Autodesk Fusion 360 part; units mm, degrees
note: some values were not read from the file. Set by a fixed rule: which face or edge a step refers to.
(part 4 of 4)
sketch "Sketch106" plane through (-154.276, 154.276, 0) normal (0.707107, -0.707107, 0) x (0.707107, 0.707107, 0)
  line L0 (-683.7427, -256.3488) -> (-383.7427, -256.3488)
  line L1 (-383.7427, -256.3488) -> (-383.7427, 273.6512)
  line L2 (-383.7427, 273.6512) -> (-683.7427, 273.6512)
  line L3 (-683.7427, 273.6512) -> (-683.7427, -256.3488)
  line L4 (-451.5546, -67.3925) -> (-616.5546, -67.3925)
  line L5 (-616.5546, -67.3925) -> (-616.5546, 97.6075)
  line L6 (-616.5546, 97.6075) -> (-451.5546, 97.6075)
  line L7 (-451.5546, 97.6075) -> (-451.5546, -67.3925)
  line L8 (-634.0546, 115.1075) -> (-434.0546, 115.1075)
  line L9 (-434.0546, 115.1075) -> (-434.0546, -84.8925)
  line L10 (-434.0546, -84.8925) -> (-634.0546, -84.8925)
  line L11 (-634.0546, -84.8925) -> (-634.0546, 115.1075)
  dimension "d553" = 200
  dimension "d554" = 200
  constraint horizontal L8
  constraint vertical L9
  constraint horizontal L10
  constraint vertical L11
  measures "d553" distance of L8.start L8.end
  measures "d554" distance of L8.start L10.end
extrude "Extrude70" cut sketch "Sketch106" against normal blind 10 contours L8 L9 L10 L11 bodies 9
sketch "Sketch107" plane through (0, -41, 0) normal (0, -1, 0) x (1, 0, 0)
  circle A0 centre (-282.6941, 15.6014) radius 82.5
  line L0 (-412.6941, -83.8986) -> (-392.6941, -103.8986)
  line L1 (-392.6941, -103.8986) -> (-172.6941, -103.8986)
  line L2 (-172.6941, -103.8986) -> (-152.6941, -83.8986)
  line L3 (-152.6941, -83.8986) -> (-152.6941, 116.1014)
  line L4 (-152.6941, 116.1014) -> (-172.6941, 136.1014)
  line L5 (-172.6941, 136.1014) -> (-392.6941, 136.1014)
  line L6 (-392.6941, 136.1014) -> (-412.6941, 116.1014)
  line L7 (-412.6941, 116.1014) -> (-412.6941, -83.8986)
  line L8 (-367.6941, 101.1014) -> (-197.6941, 101.1014)
  line L9 (-197.6941, 101.1014) -> (-197.6941, -68.8986)
  line L10 (-197.6941, -68.8986) -> (-367.6941, -68.8986)
  line L11 (-367.6941, -68.8986) -> (-367.6941, 101.1014)
  dimension "d557" = 170
  dimension "d558" = 170
  constraint horizontal L8
  constraint vertical L9
  constraint horizontal L10
  constraint vertical L11
  measures "d557" distance of L8.start L8.end
  measures "d558" distance of L8.start L10.end
extrude "Extrude71" add sketch "Sketch107" along normal blind 0.1 separate body contours A0 | L8 L9 L10 L11 makes body 34
sketch "Sketch108" plane through (0, -41, 0) normal (0, -1, 0) x (1, 0, 0)
sketch "Sketch109" plane through (0, -41, 0) normal (0, -1, 0) x (1, 0, 0)
  line L0 (-375.6941, -61.8986) -> (-367.6941, -61.8986)
  line L1 (-360.6941, -68.8986) -> (-360.6941, -76.8986)
  line L2 (-360.6941, -76.8986) -> (-375.6941, -76.8986)
  line L3 (-375.6941, -76.8986) -> (-375.6941, -61.8986)
  line L4 (-197.6941, -61.8986) -> (-189.6941, -61.8986)
  line L5 (-189.6941, -61.8986) -> (-189.6941, -76.8986)
  line L6 (-189.6941, -76.8986) -> (-204.6941, -76.8986)
  line L7 (-204.6941, -76.8986) -> (-204.6941, -68.8986)
  line L8 (-360.6941, -68.8986) -> (-367.6941, -68.8986)
  line L9 (-367.6941, -68.8986) -> (-367.6941, -61.8986)
  line L10 (-197.6941, -61.8986) -> (-197.6941, -68.8986)
  line L11 (-197.6941, -68.8986) -> (-204.6941, -68.8986)
  circle A0 centre (-193.6941, -72.8986) radius 2
  circle A1 centre (-371.6941, -72.8986) radius 2
  point P0 (-367.6941, -68.8986)
  point P1 (-197.6941, -68.8986)
  dimension "d568" = 15
  dimension "d573" = 7
  dimension "d576" = 4
  dimension "d577" = 4
  constraint horizontal L0
  constraint vertical L1
  constraint horizontal L2
  constraint vertical L3
  constraint horizontal L4
  constraint vertical L5
  constraint horizontal L6
  constraint vertical L7
  constraint horizontal L8
  constraint vertical L9
  constraint vertical L10
  constraint horizontal L11
  constraint coincident P0 L8.end
  constraint coincident P1 L10.end
  measures "d568" distance of L0.start L2.end
  measures "d573" distance of L0.end P0
  measures "d576" diameter of A0
  measures "d577" diameter of A1
extrude "Extrude72" add sketch "Sketch109" along normal blind 3 separate body makes body 35 at (-363.0274, -41, -71.5653) makes body 36 at (-202.3608, -41, -71.5653)
sketch "Sketch110" plane through (0, -38, 0) normal (0, 1, 0) x (-1, 0, 0)
sketch "Sketch111" plane through (0, -41, 0) normal (0, -1, 0) x (1, 0, 0)
  circle A0 centre (-371.6941, -72.8986) radius 2
  circle A1 centre (-193.7228, -72.9066) radius 2
  point P0 (-375.6941, -76.8986)
  point P1 (-189.6941, -76.8986)
  dimension "d580" = 4
  dimension "d581" = 4
  measures "d580" diameter of A0
  measures "d581" diameter of A1
sketch "Sketch112" plane through (0, -41, 0) normal (0, -1, 0) x (1, 0, 0)
sketch "Sketch113" plane through (0, -41, 0) normal (0, -1, 0) x (1, 0, 0)
sketch "Sketch114" plane through (0, -41, 0) normal (0, -1, 0) x (1, 0, 0)
extrude "Extrude73" cut sketch "Sketch111" against normal blind 3 bodies 30
sketch "Sketch115" plane through (0, 0, 273.1014) normal (0, 0, 1) x (-1, 0, 0)
  arc A0 (177.6941, 0) -> (172.6941, 0) centre (175.1941, 0) ccw
  line L0 (177.6941, 0) -> (197.6941, 0)
  arc A1 (202.6941, 0) -> (197.6941, 0) centre (200.1941, 0) ccw
  line L1 (202.6941, 0) -> (202.6941, -10)
  line L2 (202.6941, -10) -> (362.6941, -10)
  line L3 (362.6941, -10) -> (362.6941, 0)
  arc A2 (367.694, 0) -> (362.6941, 0) centre (365.1941, 0.0132) ccw
  line L4 (367.694, 0) -> (387.6941, 0)
  arc A3 (392.6941, 0) -> (387.6941, 0) centre (390.1941, 0) ccw
  line L5 (392.6941, 0) -> (392.6941, -10)
  line L6 (392.6941, -10) -> (422.6941, -10)
  line L7 (422.6941, -10) -> (422.6941, 25)
  arc A4 (422.6941, 30) -> (422.6941, 25) centre (422.6941, 27.5) ccw
  line L8 (422.6941, 30) -> (432.6941, 30)
  line L9 (432.6941, 30) -> (432.6941, 60)
  line L10 (432.6941, 60) -> (422.6941, 60)
  arc A5 (422.6941, 65) -> (422.6941, 60) centre (422.6941, 62.5) ccw
  line L11 (422.6941, 65) -> (422.6941, 100)
  line L12 (422.6941, 100) -> (142.6941, 100)
  line L13 (142.6941, 100) -> (142.6941, 65)
  arc A6 (142.6941, 60) -> (142.6941, 65) centre (142.6941, 62.5) ccw
  line L14 (142.6941, 60) -> (132.6941, 60)
  line L15 (132.6941, 60) -> (132.6941, 30)
  line L16 (132.6941, 30) -> (142.6941, 30)
  arc A7 (142.6941, 25) -> (142.6941, 30) centre (142.6941, 27.5) ccw
  line L17 (142.6941, 25) -> (142.6941, -10)
  line L18 (142.6941, -10) -> (172.6941, -10)
  line L19 (172.6941, -10) -> (172.6941, 0)
  circle A8 centre (400.1941, 22.3451) radius 12.5
sketch "Sketch116" plane through (0, 0, -256.8986) normal (0, 0, -1) x (1, 0, 0)
  line L0 (-332.6941, 30) -> (-332.6941, 80)
  line L1 (-332.6941, 80) -> (-232.6941, 80)
  line L2 (-232.6941, 80) -> (-232.6941, 30)
  line L3 (-232.6941, 30) -> (-332.6941, 30)
  arc A0 (-172.6941, 0) -> (-177.6941, 0) centre (-175.1941, 0) ccw
  line L4 (-172.6941, 0) -> (-172.6941, -10)
  line L5 (-172.6941, -10) -> (-142.6941, -10)
  line L6 (-142.6941, -10) -> (-142.6941, 25)
  arc A1 (-142.6941, 30) -> (-142.6941, 25) centre (-142.6941, 27.5) ccw
  line L7 (-142.6941, 30) -> (-132.6941, 30)
  line L8 (-132.6941, 30) -> (-132.6941, 60)
  line L9 (-132.6941, 60) -> (-142.6941, 60)
  arc A2 (-142.6941, 65) -> (-142.6941, 60) centre (-142.6941, 62.5) ccw
  line L10 (-142.6941, 65) -> (-142.6941, 100)
  line L11 (-142.6941, 100) -> (-422.6941, 100)
  line L12 (-422.6941, 100) -> (-422.6941, 65)
  arc A3 (-422.6941, 60) -> (-422.6941, 65) centre (-422.6941, 62.5) ccw
  line L13 (-422.6941, 60) -> (-432.6941, 60)
  line L14 (-432.6941, 60) -> (-432.6941, 30)
  line L15 (-432.6941, 30) -> (-422.6941, 30)
  arc A4 (-422.6941, 25) -> (-422.6941, 30) centre (-422.6941, 27.5) ccw
  line L16 (-422.6941, 25) -> (-422.6941, -10)
  line L17 (-422.6941, -10) -> (-392.6941, -10)
  line L18 (-392.6941, -10) -> (-392.6941, 0)
  arc A5 (-387.6941, 0) -> (-392.6941, 0) centre (-390.1941, 0) ccw
  line L19 (-387.6941, 0) -> (-367.694, 0)
  arc A6 (-362.6941, 0) -> (-367.694, 0) centre (-365.1941, 0.0132) ccw
  line L20 (-362.6941, 0) -> (-362.6941, -10)
  line L21 (-362.6941, -10) -> (-202.6941, -10)
  line L22 (-202.6941, -10) -> (-202.6941, 0)
  arc A7 (-197.6941, 0) -> (-202.6941, 0) centre (-200.1941, 0) ccw
  line L23 (-197.6941, 0) -> (-177.6941, 0)
  circle A8 centre (-407.6941, 15.2463) radius 10
  dimension "d591" = 20
  measures "d591" diameter of A8
extrude "Extrude75" cut sketch "Sketch116" against normal blind 10 contours A8 bodies 8
move_body "Move26" bodies 34 to x (1, 0, 0) y (0, 1, 0) z (0, 0, 1) at (0, -0.5, 0)
sketch "Sketch117" plane through (-222.6941, 0, 0) normal (1, 0, 0) x (0, 1, 0)
  arc A0 (0, 203.1014) -> (0, 198.1014) centre (0, 200.6014) ccw
  line L0 (0, 203.1014) -> (0, 213.1014)
  line L1 (0, 213.1014) -> (-60, 213.1014)
  arc A1 (-65, 213.1014) -> (-60, 213.1014) centre (-62.5, 213.1014) ccw
  line L2 (-65, 213.1014) -> (-65, 223.1014)
  line L3 (-65, 223.1014) -> (-70, 223.1014)
  line L4 (-70, 223.1014) -> (-70, 190)
  line L5 (-70, 190) -> (-5.4259, 163.1014)
  line L6 (-5.4259, 163.1014) -> (0, 163.1014)
  line L7 (0, 163.1014) -> (0, 173.1014)
  arc A2 (0, 178.1014) -> (0, 173.1014) centre (0, 175.6014) ccw
  line L8 (0, 178.1014) -> (10, 178.1014)
  line L9 (10, 178.1014) -> (10, 198.1014)
  line L10 (10, 198.1014) -> (0, 198.1014)
  line L11 (-43.0336, 296.8431) -> (-76.8948, 279.4893)
  circle A3 centre (1.9664, 213.1014) radius 45
  circle A4 centre (1.9664, 213.1014) radius 4
  dimension "d594" = 38.0492
  dimension "d597" = 90
  dimension "d598" = 8
  constraint concentric A3 A4
  measures "d594" distance of L11.start L11.end
  measures "d597" diameter of A3
  measures "d598" diameter of A4
extrude "Extrude76" add sketch "Sketch117" against normal blind 90 separate body contours A0 L0 L1 L7 A2 L8 L9 L10 A3 A4 | A0 L0 L1 L7 A2 L8 L9 L10 A3 A4 makes body 37
move_body "Move27" bodies 37 to x (1, 0, 0) y (0, 1, 0) z (0, 0, 1) at (-15, 0, 0)
sketch "Sketch118" plane through (0, 0, 0) normal (0, 1, 0) x (1, 0, 0)
sketch "Sketch119" plane through (-237.6941, 0, 0) normal (1, 0, 0) x (0, 1, 0)
  circle A0 centre (1.9664, 213.1014) radius 4
  circle A1 centre (1.9664, 213.1014) radius 45
sketch "Sketch120" plane through (-237.6941, 1.9664, 213.1014) normal (1, 0, 0) x (0, 1, 0)
  line L0 (-45, 0) -> (-45, -350)
  dimension "d604" = 45
  dimension "d605" = 350
  measures "d604" distance of origin L0.start
  measures "d605" distance of L0.start L0.end
surface "Extrude77" add extruded along (1, 0, 0) between 0 and -90 path "Sketch120" along L0 separate body makes body 38
move_body "Move28" bodies 10 11 12 13 14 15 16 17 19 20 21 22 23 24 to x (1, 0, 0) y (0, 1, 0) z (0, 0, 1) at (-20, 0, 0)
move_body "Move29" bodies 34 to x (1, 0, 0) y (0, 1, 0) z (0, 0, 1) at (0, 2, 0)
move_body "Move30" bodies 38 37 to x (1, 0, 0) y (0, 1, 0) z (0, 0, 1) at (0, 4, 0)
move_body "Move31" bodies 34 to x (1, 0, 0) y (0, 1, 0) z (0, 0, 1) at (0, -2, 0)
move_body "Move32" bodies 37 38 to x (1, 0, 0) y (0, 1, 0) z (0, 0, 1) at (0, -2.1, 0)
move_body "Move33" bodies 12 13 10 to x (1, 0, 0) y (0, 1, 0) z (0, 0, 1) at (5, 0, 0)
sketch "Sketch121" plane through (0, -41, 0) normal (0, -1, 0) x (1, 0, 0)
  circle A0 centre (-371.6941, -72.8986) radius 2
  circle A1 centre (-193.7228, -72.9066) radius 2
  circle A2 centre (-282.6941, 15.6014) radius 82.5
  line L0 (-412.6941, -83.8986) -> (-392.6941, -103.8986)
  line L1 (-392.6941, -103.8986) -> (-172.6941, -103.8986)
  line L2 (-172.6941, -103.8986) -> (-152.6941, -83.8986)
  line L3 (-152.6941, -83.8986) -> (-152.6941, 116.1014)
  line L4 (-152.6941, 116.1014) -> (-172.6941, 136.1014)
  line L5 (-172.6941, 136.1014) -> (-392.6941, 136.1014)
  line L6 (-392.6941, 136.1014) -> (-412.6941, 116.1014)
  line L7 (-412.6941, 116.1014) -> (-412.6941, -83.8986)
sketch "Sketch122" plane through (0, -41.1336, 0) normal (0, 1, 0) x (-1, 0, 0)
  line L0 (237.6941, 213.1014) -> (237.6941, -136.8986)
  line L1 (237.6941, -136.8986) -> (327.6941, -136.8986)
  line L2 (327.6941, -136.8986) -> (327.6941, 213.1014)
  line L3 (327.6941, 213.1014) -> (237.6941, 213.1014)
sketch "Sketch123" plane through (0, -41.1336, 0) normal (0, 1, 0) x (-1, 0, 0)
sketch "Sketch124" plane through (0, -41.1336, 0) normal (0, 1, 0) x (-1, 0, 0)
move_face "MoveFace5" to x (1, 0, 0) y (0, 1, 0) z (0, 0, 1) at (1, 0, 0) 1 faces at (-267.6941, -40.91, 217.5819) on bodies 37
move_body "Move34" bodies 38 to x (1, 0, 0) y (0, 1, 0) z (0, 0, 1) at (1, 0, 0)
move_face "MoveFace6" to x (1, 0, 0) y (0, 1, 0) z (0, 0, 1) at (1, 0, 0) 1 faces at (-267.6941, -40.91, 217.5819) on bodies 37
move_face "MoveFace7" to x (1, 0, 0) y (0, 1, 0) z (0, 0, 1) at (2, 0, 0) 1 faces at (-267.6941, -40.91, 217.5819) on bodies 37
sketch "Sketch125" plane through (-237.6941, 0, 0) normal (1, 0, 0) x (0, 1, 0)
extrude "Extrude78" add sketch "Sketch119" along normal blind -115 and the other way blind 15 separate body contours A0 makes body 39
extrude "Extrude79" add 1 faces at (-252.6941, 3.0166, 214.9798) along direction (1, 0, 0) blind 40 on bodies 39 bodies 39 6
delete_face "DeleteFace1" 2 faces at (-319.3608, -1.7195, 211.5476) (-232.6941, -2.0138, 213.4996) on bodies 39
move_face "MoveFace8" by (0, 0, 4) 1 faces at (-237.6941, 35.0322, 210.8657) on bodies 37
move_body "Move35" bodies 37 to x (1, 0, 0) y (0, 1, 0) z (0, 0, 1) at (0, -8, 4)
sketch "Sketch126" plane through (-237.6941, 0, 0) normal (1, 0, 0) x (0, 1, 0)
  circle A0 centre (-4.1336, 217.1014) radius 4
  circle A1 centre (-4.1336, 217.1014) radius 45
  circle A2 centre (-4.1336, 217.1014) radius 4
  dimension "d615" = 8
  constraint concentric A0 A2
  measures "d615" diameter of A2
extrude "Extrude80" add sketch "Sketch126" along normal blind -115 and the other way blind -20 separate body contours A0 A2 makes body 40
move_body "Move36" bodies 40 to x (1, 0, 0) y (0, 1, 0) z (0, 0, 1) at (5, 0, 0)
extrude "Extrude74" [suppressed]
sketch "Sketch82" plane through (-206.2361, 0, 0) normal (1, 0, 0) x (0, 1, 0)
  line L0 (-51.8339, -133.2604) -> (-39.3469, -133.2411)
  line L1 (-39.3469, -139.2411) -> (-51.4948, -139.2411)
  arc A0 (-51.1648, -133.2593) -> (-51.4948, -139.2411) centre (-51.4948, -136.2411) ccw
  arc A1 (-39.3469, -139.2411) -> (-39.3469, -133.2411) centre (-39.3423, -136.2411) ccw
  dimension "d390" = 6
  dimension "d391" = 6
  constraint coincident L0.start A0
  constraint tangent L0 A1
  constraint tangent L1 A0
  constraint coincident L0 A0.start
  measures "d390" diameter of A1
  measures "d391" diameter of A0
extrude "Extrude15" [suppressed]
sketch "Sketch30" plane through (0, 0, 0) normal (0, -1, 0) x (1, 0, 0)
sketch "Sketch31" plane through (0, 0, 0) normal (1, 0, 0) x (0, 1, 0)
sketch "Sketch32" plane through (-132.6941, 0, 0) normal (1, 0, 0) x (0, 1, 0)
  line L0 (0, 140.6014) -> (0, 150.6014)
  arc A0 (0, 155.6014) -> (0, 150.6014) centre (0, 153.1014) ccw
  line L1 (0, 155.6014) -> (10, 155.6014)
  line L2 (10, 155.6014) -> (10, 273.6512)
  line L3 (10, 273.6512) -> (-30, 273.6512)
  line L4 (-30, 273.6512) -> (-30, 263.6512)
  arc A1 (-35, 263.6512) -> (-30, 263.6512) centre (-32.5, 263.6512) ccw
  line L5 (-35, 263.6512) -> (-55, 263.6512)
  arc A2 (-60, 263.6512) -> (-55, 263.6512) centre (-57.5, 263.6512) ccw
  line L6 (-60, 263.6512) -> (-60, 273.6512)
  line L7 (-60, 273.6512) -> (-100, 273.6512)
  line L8 (-100, 273.6512) -> (-100, -256.3488)
  line L9 (-100, -256.3488) -> (-60, -256.3488)
  line L10 (-60, -256.3488) -> (-60, -246.3488)
  arc A3 (-55, -246.3488) -> (-60, -246.3488) centre (-57.5, -246.3488) ccw
  line L11 (-55, -246.3488) -> (-35, -246.3488)
  arc A4 (-30, -246.3488) -> (-35, -246.3488) centre (-32.5, -246.3488) ccw
  line L12 (-30, -246.3488) -> (-30, -256.3488)
  line L13 (-30, -256.3488) -> (10, -256.3488)
  line L14 (10, -256.3488) -> (10, -149.3986)
  line L15 (10, -149.3986) -> (0, -149.3986)
  arc A5 (0, -144.3986) -> (0, -149.3986) centre (0, -146.8986) ccw
  line L16 (0, -144.3986) -> (0, -124.3986)
  arc A6 (0, -119.3986) -> (0, -124.3986) centre (0, -121.8986) ccw
  line L17 (0, -119.3986) -> (10, -119.3986)
  line L18 (10, -119.3986) -> (10, -11.8986)
  line L19 (10, -11.8986) -> (0, -11.8986)
  arc A7 (0, -6.8986) -> (0, -11.8986) centre (0, -9.3986) ccw
  line L20 (0, -6.8986) -> (0, 13.1014)
  arc A8 (0, 18.1014) -> (0, 13.1014) centre (0, 15.6014) ccw
  line L21 (0, 18.1014) -> (10, 18.1014)
  line L22 (10, 18.1014) -> (10, 125.6014)
  line L23 (10, 125.6014) -> (0, 125.6014)
  arc A9 (0, 130.6014) -> (0, 125.6014) centre (0, 128.1014) ccw
  line L24 (0, 130.6014) -> (0, 135.6014)
  arc A10 (0, 140.6014) -> (0, 135.6014) centre (0, 138.1014) ccw
  circle A11 centre (-25, -180) radius 4
  circle A12 centre (-50, 175) radius 4
  circle A13 centre (-25, 170) radius 4
  circle A14 centre (-50, -175) radius 4
  circle A15 centre (-75, 180) radius 4
  circle A16 centre (-75, -170) radius 4
  line L25 (-6, 141.6014) -> (0, 141.6014)
  line L26 (0, 141.6014) -> (0, 135.6014)
  line L27 (0, 135.6014) -> (-6, 135.6014)
  line L28 (-6, 135.6014) -> (-6, 141.6014)
  dimension "d219" = 6
  dimension "d220" = 6
  constraint horizontal L25
  constraint vertical L26
  constraint horizontal L27
  constraint vertical L28
  constraint coincident L24.end A10.end
  measures "d219" distance of L25.start L25.end
  measures "d220" distance of L25.start L27.end
sketch "Sketch33" plane through (-132.6941, 0, 0) normal (1, 0, 0) x (0, 1, 0)
  line L0 (0, 140.6014) -> (0, 150.6014)
  arc A0 (0, 155.6014) -> (0, 150.6014) centre (0, 153.1014) ccw
  line L1 (0, 155.6014) -> (10, 155.6014)
  line L2 (10, 155.6014) -> (10, 273.6512)
  line L3 (10, 273.6512) -> (-30, 273.6512)
  line L4 (-30, 273.6512) -> (-30, 263.6512)
  arc A1 (-35, 263.6512) -> (-30, 263.6512) centre (-32.5, 263.6512) ccw
  line L5 (-35, 263.6512) -> (-55, 263.6512)
  arc A2 (-60, 263.6512) -> (-55, 263.6512) centre (-57.5, 263.6512) ccw
  line L6 (-60, 263.6512) -> (-60, 273.6512)
  line L7 (-60, 273.6512) -> (-100, 273.6512)
  line L8 (-100, 273.6512) -> (-100, -256.3488)
  line L9 (-100, -256.3488) -> (-60, -256.3488)
  line L10 (-60, -256.3488) -> (-60, -246.3488)
  arc A3 (-55, -246.3488) -> (-60, -246.3488) centre (-57.5, -246.3488) ccw
  line L11 (-55, -246.3488) -> (-35, -246.3488)
  arc A4 (-30, -246.3488) -> (-35, -246.3488) centre (-32.5, -246.3488) ccw
  line L12 (-30, -246.3488) -> (-30, -256.3488)
  line L13 (-30, -256.3488) -> (10, -256.3488)
  line L14 (10, -256.3488) -> (10, -149.3986)
  line L15 (10, -149.3986) -> (0, -149.3986)
  arc A5 (0, -144.3986) -> (0, -149.3986) centre (0, -146.8986) ccw
  line L16 (0, -144.3986) -> (0, -124.3986)
  arc A6 (0, -119.3986) -> (0, -124.3986) centre (0, -121.8986) ccw
  line L17 (0, -119.3986) -> (10, -119.3986)
  line L18 (10, -119.3986) -> (10, -11.8986)
  line L19 (10, -11.8986) -> (0, -11.8986)
  arc A7 (0, -6.8986) -> (0, -11.8986) centre (0, -9.3986) ccw
  line L20 (0, -6.8986) -> (0, 13.1014)
  arc A8 (0, 18.1014) -> (0, 13.1014) centre (0, 15.6014) ccw
  line L21 (0, 18.1014) -> (10, 18.1014)
  line L22 (10, 18.1014) -> (10, 125.6014)
  line L23 (10, 125.6014) -> (0, 125.6014)
  arc A9 (0, 130.6014) -> (0, 125.6014) centre (0, 128.1014) ccw
  line L24 (0, 130.6014) -> (0, 135.6014)
  arc A10 (0, 140.6014) -> (0, 135.6014) centre (0, 138.1014) ccw
  circle A11 centre (-25, -180) radius 4
  circle A12 centre (-50, 175) radius 4
  circle A13 centre (-25, 170) radius 4
  circle A14 centre (-50, -175) radius 4
  circle A15 centre (-75, 180) radius 4
  circle A16 centre (-75, -170) radius 4
  line L25 (0, 135.6014) -> (0, 138.6108)
  constraint vertical L25
  constraint coincident L24.end A10.end
sketch "Sketch34" plane through (-132.6941, 0, 0) normal (1, 0, 0) x (0, 1, 0)
  line L0 (9.8069, 125.4872) -> (-5.1931, 125.4872)
  line L1 (-5.1931, 125.4872) -> (-5.1931, 155.4872)
  line L2 (-5.1931, 155.4872) -> (9.8069, 155.4872)
  line L3 (9.8069, 155.4872) -> (9.8069, 125.4872)
  dimension "d225" = 15
  dimension "d226" = 30
  constraint horizontal L0
  constraint vertical L1
  constraint horizontal L2
  constraint vertical L3
  measures "d225" distance of L0.start L0.end
  measures "d226" distance of L0.start L2.end
sketch "Sketch35" plane through (-422.6941, 0, 0) normal (1, 0, 0) x (0, 1, 0)
  circle A0 centre (-75, -170) radius 4
  circle A1 centre (-75, 180) radius 4
  circle A2 centre (-50, -175) radius 4
  circle A3 centre (-25, 170) radius 4
  circle A4 centre (-50, 175) radius 4
  circle A5 centre (-25, -180) radius 4
  arc A6 (0, 115.6014) -> (0, 110.6014) centre (0, 113.1014) ccw
  line L0 (0, 115.6014) -> (0, 135.6014)
  arc A7 (0, 140.6014) -> (0, 135.6014) centre (0, 138.1014) ccw
  line L1 (0, 140.6014) -> (10, 140.6014)
  line L2 (10, 140.6014) -> (10, 273.6512)
  line L3 (10, 273.6512) -> (-30, 273.6512)
  line L4 (-30, 273.6512) -> (-30, 263.6512)
  arc A8 (-35, 263.6512) -> (-30, 263.6512) centre (-32.5, 263.6512) ccw
  line L5 (-35, 263.6512) -> (-55, 263.6512)
  arc A9 (-60, 263.6512) -> (-55, 263.6512) centre (-57.5, 263.6512) ccw
  line L6 (-60, 263.6512) -> (-60, 273.6512)
  line L7 (-60, 273.6512) -> (-100, 273.6512)
  line L8 (-100, 273.6512) -> (-100, -256.3488)
  line L9 (-100, -256.3488) -> (-60, -256.3488)
  line L10 (-60, -256.3488) -> (-60, -246.3488)
  arc A10 (-55, -246.3488) -> (-60, -246.3488) centre (-57.5, -246.3488) ccw
  line L11 (-55, -246.3488) -> (-35, -246.3488)
  arc A11 (-30, -246.3488) -> (-35, -246.3488) centre (-32.5, -246.3488) ccw
  line L12 (-30, -246.3488) -> (-30, -256.3488)
  line L13 (-30, -256.3488) -> (10, -256.3488)
  line L14 (10, -256.3488) -> (10, -149.3986)
  line L15 (10, -149.3986) -> (0, -149.3986)
  arc A12 (0, -144.3986) -> (0, -149.3986) centre (0, -146.8986) ccw
  line L16 (0, -144.3986) -> (0, -124.3986)
  arc A13 (0, -119.3986) -> (0, -124.3986) centre (0, -121.8986) ccw
  line L17 (0, -119.3986) -> (10, -119.3986)
  line L18 (10, -119.3986) -> (10, -11.8986)
  line L19 (10, -11.8986) -> (0, -11.8986)
  arc A14 (0, -6.8986) -> (0, -11.8986) centre (0, -9.3986) ccw
  line L20 (0, -6.8986) -> (0, 13.1014)
  arc A15 (0, 18.1014) -> (0, 13.1014) centre (0, 15.6014) ccw
  line L21 (0, 18.1014) -> (10, 18.1014)
  line L22 (10, 18.1014) -> (10, 110.6014)
  line L23 (10, 110.6014) -> (0, 110.6014)
  line L24 (62.048, 125) -> (72.048, 125)
  line L25 (72.048, 125) -> (72.048, 155)
  line L26 (72.048, 155) -> (62.048, 155)
  line L27 (62.048, 155) -> (62.048, 125)
  line L28 (10, 140.6014) -> (10, 110.6014)
  dimension "d227" = 10
  dimension "d228" = 30
  constraint horizontal L24
  constraint vertical L25
  constraint horizontal L26
  constraint vertical L27
  constraint coincident L1.end L2.start
  constraint coincident L22.end L23.start
  measures "d227" distance of L24.start L24.end
  measures "d228" distance of L24.start L26.end
extrude "Extrude16" [suppressed]
sketch "Sketch15" plane through (-132.6941, 0, 0) normal (1, 0, 0) x (0, 1, 0)
  arc A0 (0, 115.6014) -> (0, 110.6014) centre (0, 113.1014) ccw
  line L0 (0, 115.6014) -> (0, 135.6014)
  arc A1 (0, 140.6014) -> (0, 135.6014) centre (0, 138.1014) ccw
  line L1 (0, 140.6014) -> (10, 140.6014)
  line L2 (10, 140.6014) -> (10, 273.6512)
  line L3 (10, 273.6512) -> (-30, 273.6512)
  line L4 (-30, 273.6512) -> (-30, 263.6512)
  arc A2 (-35, 263.6512) -> (-30, 263.6512) centre (-32.5, 263.6512) ccw
  line L5 (-35, 263.6512) -> (-55, 263.6512)
  arc A3 (-60, 263.6512) -> (-55, 263.6512) centre (-57.5, 263.6512) ccw
  line L6 (-60, 263.6512) -> (-60, 273.6512)
  line L7 (-60, 273.6512) -> (-100, 273.6512)
  line L8 (-100, 273.6512) -> (-100, -256.3488)
  line L9 (-100, -256.3488) -> (-60, -256.3488)
  line L10 (-60, -256.3488) -> (-60, -246.3488)
  arc A4 (-55, -246.3488) -> (-60, -246.3488) centre (-57.5, -246.3488) ccw
  line L11 (-55, -246.3488) -> (-35, -246.3488)
  arc A5 (-30, -246.3488) -> (-35, -246.3488) centre (-32.5, -246.3488) ccw
  line L12 (-30, -246.3488) -> (-30, -256.3488)
  line L13 (-30, -256.3488) -> (10, -256.3488)
  line L14 (10, -256.3488) -> (10, -149.3986)
  line L15 (10, -149.3986) -> (0, -149.3986)
  arc A6 (0, -144.3986) -> (0, -149.3986) centre (0, -146.8986) ccw
  line L16 (0, -144.3986) -> (0, -124.3986)
  arc A7 (0, -119.3986) -> (0, -124.3986) centre (0, -121.8986) ccw
  line L17 (0, -119.3986) -> (10, -119.3986)
  line L18 (10, -119.3986) -> (10, -11.8986)
  line L19 (10, -11.8986) -> (0, -11.8986)
  arc A8 (0, -6.8986) -> (0, -11.8986) centre (0, -9.3986) ccw
  line L20 (0, -6.8986) -> (0, 13.1014)
  arc A9 (0, 18.1014) -> (0, 13.1014) centre (0, 15.6014) ccw
  line L21 (0, 18.1014) -> (10, 18.1014)
  line L22 (10, 18.1014) -> (10, 110.6014)
  line L23 (10, 110.6014) -> (0, 110.6014)
sketch "Sketch16" plane through (-132.6941, 0, 0) normal (1, 0, 0) x (0, 1, 0)
  circle A0 centre (-75, 250) radius 4
  dimension "d145" = 8
  measures "d145" diameter of A0
sketch "Sketch17" plane through (-132.6941, 0, 0) normal (1, 0, 0) x (0, 1, 0)
  circle A0 centre (-75, 250) radius 4
  circle A1 centre (-50, 245) radius 4
  circle A2 centre (-25, 240) radius 4
  dimension "d148" = 8
  dimension "d149" = 8
  dimension "d150" = 8
  measures "d148" diameter of A0
  measures "d149" diameter of A1
  measures "d150" diameter of A2
extrude "Extrude4" [suppressed]
sketch "Sketch18" plane through (-132.6941, 0, 0) normal (1, 0, 0) x (0, 1, 0)
sketch "Sketch6" plane through (0, 0, 0) normal (0, 1, 0) x (1, 0, 0)
  line L0 (-130.6524, -417.4507) -> (149.3476, -417.4507)
  line L1 (149.3476, -417.4507) -> (149.3476, 102.5493)
  line L2 (149.3476, 102.5493) -> (-130.6524, 102.5493)
  line L3 (-130.6524, 102.5493) -> (-130.6524, -417.4507)
  line L4 (-70.6524, -417.4507) -> (89.3476, -417.4507)
  line L5 (89.3476, -417.4507) -> (89.3476, -257.4507)
  line L6 (89.3476, -257.4507) -> (-70.6524, -257.4507)
  line L7 (-70.6524, -257.4507) -> (-70.6524, -417.4507)
  dimension "d20" = 280
  dimension "d21" = 520
  dimension "d22" = 160
  dimension "d23" = 160
  constraint horizontal L0
  constraint vertical L1
  constraint horizontal L2
  constraint vertical L3
  constraint horizontal L4
  constraint vertical L5
  constraint horizontal L6
  constraint vertical L7
  constraint midpoint L0 L4
  measures "d20" distance of L0.start L0.end
  measures "d21" distance of L0.start L2.end
  measures "d22" distance of L4.start L4.end
  measures "d23" distance of L4.start L6.end
sketch "Sketch7" plane through (9.3476, 0, 337.4507) normal (0, 1, 0) x (1, 0, 0)
sketch "Sketch1 (2)" plane through (0, 0, 0) normal (0, 1, 0) x (1, 0, 0)
  line L0 (-365.8238, -74.8534) -> (-365.8238, 442.7199)
  line L1 (-365.8238, 442.7199) -> (-47.879, 442.7199)
  line L2 (-290.6781, 85.8869) -> (-125.6781, 85.8869)
  line L3 (-125.6781, 85.8869) -> (-125.6781, 250.8869)
  line L4 (-125.6781, 250.8869) -> (-290.6781, 250.8869)
  line L5 (-290.6781, 250.8869) -> (-290.6781, 85.8869)
  line L6 (-65.9448, -83.3727) -> (-65.9448, 85.8869)
  line L7 (-365.8238, 90.1466) -> (-365.8238, -74.8534)
  line L8 (-348.1781, 440) -> (-365.8238, 440)
  line L9 (-365.8238, 440) -> (-365.8238, -74.8534)
  line L10 (-65.8313, -76.9701) -> (-75.8313, -76.9701)
  line L11 (-68.1781, 440.8869) -> (-65.8313, 440.8869)
  line L12 (-65.8313, 440.8869) -> (-65.8313, -76.9701)
  line L13 (-365.8238, -74.8534) -> (-345.8238, -74.8534)
  line L14 (-345.8238, -74.8534) -> (-65.9448, -83.3727)
  line L15 (-255.8843, -79.1131) -> (-155.8843, -79.1131)
  line L16 (-155.8843, -79.1131) -> (-155.8843, 20.8869)
  line L17 (-155.8843, 20.8869) -> (-255.8843, 20.8869)
  line L18 (-255.8843, 20.8869) -> (-255.8843, -79.1131)
  line L19 (-365.8238, -74.8534) -> (-355.8238, -74.8534)
  line L20 (-348.1781, -594.8384) -> (-361.8683, -594.8384)
  dimension "d1" = 300
  dimension "d2" = 520
  dimension "d3" = 165
  dimension "d4" = 165
  dimension "d5" = 300
  dimension "d6" = 165
  dimension "d8" = 10
  dimension "d13" = 100
  dimension "d14" = 100
  dimension "d15" = 10
  dimension "d16" = 520
  constraint vertical L0
  constraint horizontal L1
  constraint horizontal L2
  constraint vertical L3
  constraint horizontal L4
  constraint vertical L5
  constraint vertical L6
  constraint vertical L7
  constraint horizontal L8
  constraint vertical L9
  constraint horizontal L10
  constraint horizontal L11
  constraint vertical L12
  constraint perpendicular L0 L13
  constraint horizontal L15
  constraint vertical L16
  constraint horizontal L17
  constraint vertical L18
  constraint midpoint L14 L15
  constraint horizontal L19
  constraint horizontal L20
  measures "d1" distance of L10.start L0.start
  measures "d2" distance of L10.start L1.end
  measures "d3" distance of L2.start L2.end
  measures "d4" distance of L2.start L4.end
  measures "d5" distance of L0.start L6.start
  measures "d6" distance of L0.start L7.start
  measures "d8" distance of L10.start L10.end
  measures "d13" distance of L15.start L15.end
  measures "d14" distance of L15.start L17.end
  measures "d15" distance of L0.start L19.end
  measures "d16" distance of L0.start L20.end
sketch "Sketch2 (2)" plane through (0, 0, 0) normal (0, 1, 0) x (1, 0, 0)
  line L0 (-360, -80) -> (-40, -80)
  line L1 (-40, -80) -> (-40, -30)
  line L2 (-40, -30) -> (-360, -30)
  line L3 (-360, -30) -> (-360, -80)
  line L4 (-360, 440) -> (-30, 440)
  line L5 (-30, 440) -> (-30, 390)
  line L6 (-30, 390) -> (-360, 390)
  line L7 (-360, 390) -> (-360, 440)
  line L8 (-360, -30) -> (-20, -30)
  line L9 (-20, -30) -> (-20, 120)
  line L10 (-20, 120) -> (-360, 120)
  line L11 (-360, 120) -> (-360, -30)
  line L12 (-360, 390) -> (-20, 390)
  line L13 (-20, 390) -> (-20, 240)
  line L14 (-20, 240) -> (-360, 240)
  line L15 (-360, 240) -> (-360, 390)
  line L16 (-68.1292, -30) -> (-57.9852, -30)
  line L17 (-57.9852, -30) -> (-57.9852, 0)
  line L18 (-57.9852, 0) -> (-68.1292, 0)
  line L19 (-68.1292, 0) -> (-68.1292, -30)
  dimension "d17" = 50
  constraint horizontal L0
  constraint vertical L1
  constraint horizontal L2
  constraint vertical L3
  constraint horizontal L4
  constraint vertical L5
  constraint horizontal L6
  constraint vertical L7
  constraint horizontal L8
  constraint vertical L9
  constraint horizontal L10
  constraint vertical L11
  constraint horizontal L12
  constraint vertical L13
  constraint horizontal L14
  constraint vertical L15
  constraint horizontal L16
  constraint vertical L17
  constraint horizontal L18
  constraint vertical L19
  constraint coincident L2 L16.start
  measures "d17" distance of L0.start L2.end
sketch "Sketch3 (2)" plane through (0, 0, 0) normal (0, 1, 0) x (1, 0, 0)
sketch "Sketch4" plane through (0, 0, 0) normal (0, 1, 0) x (-1, 0, 0)
sketch "Sketch5" plane through (0, 0, 0) normal (0, 1, 0) x (1, 0, 0)
  circle A0 centre (-68, -32.5) radius 2.2636
  circle A1 centre (-68, 2.5) radius 2.5
component "Side" placed x (1, 0, 0) y (0, 1, 0) z (0, 0, 1) at (0, 0, 0)
equation "d457 = d456"
equation "d459 = d458"
equation "d461 = d460"
equation "d463 = d462"
named bodies: "Base Plate", "Right Panel", "Side Plate", "Left Panel", "Spacer", "Left Paper Mount", "Right Paper Mount", "Top", "Bottom", "Door", "Motor Base Plate", "Right Paper Plate", "Gear Motor", "Motor Mount", "Drive Shaft", "Left Paper Plate", "Left Spring Cap", "Right Spring Cap", "Idler Shaft", "Idler Roller 5", "Idler Roller", "Idler Roller 1", "Idler Roller (1)", "Idler Roller 3", "Idler Roller (2)", "Idler Roller 4", "Idler Roller (1) (1)", "Idler Roller 2", "Sensor Frame", "East", "South", "North", "West", "Face Plate", "Left Paper Guide", "Right Paper Guide", "Paper Guide", "Target", "Left Target Guide", "Right Target Guide", "Paper Roll", "Witness Paper", "Paper Axle"
